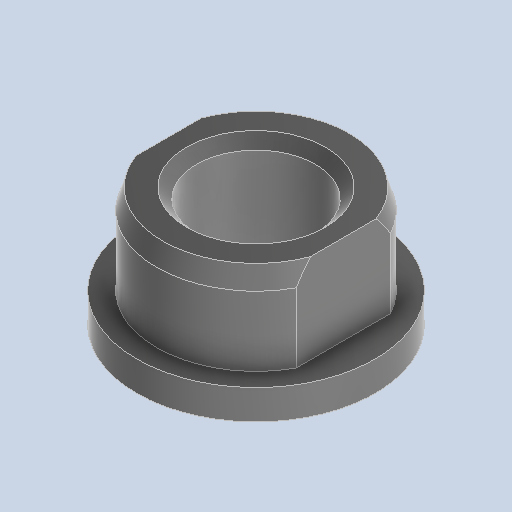
# Autodesk Inventor part: LED-0606
Saved by Autodesk Inventor 2024.2 (Build 282272000, 272)
## iProperties
Created: 2024-01-03
Part Number: LED-0606
Material: Acetal Resin, Black
Document SubType Name: Modeling
Designer: Masato Kubotera
Density: 1.425 g/cm^3
Appearance: Smooth - Black
Catalog Web Link: https://jp.misumi-ec.com/vona2/detail/221000090992/?ProductCode=LED-0606
Vendor: OILES
Mass: 0.469493 g
Surface Area: 4.64015 cm^2
Volume: 0.329469 cm^3
Author: Masato Kubotera
Autodesk Inventor part; units mm, degrees
ref_plane "YZ Plane" through (0, 0, 0) normal (1, 0, 0) x (0, 1, 0)
ref_plane "XZ Plane" through (0, 0, 0) normal (0, 1, 0) x (-1, 0, 0)
ref_plane "XY Plane" through (0, 0, 0) normal (0, 0, 1) x (1, 0, 0)
sketch "Sketch1" plane through (0, 0, 0) normal (0, 1, 0) x (-1, 0, 0)
  line L0 (0, 0) -> (0, 6)
  line L1 (-3, 0) -> (-3, 6)
  line L2 (-3, 6) -> (-5, 6)
  line L3 (-5, 6) -> (-5, 1.5)
  line L4 (-5, 1.5) -> (-6, 1.5)
  line L5 (-6, 1.5) -> (-6, 0)
  line L6 (-6, 0) -> (-3, 0)
  dimension "InsideDiameter" = 6
  dimension "OuterDiameter" = 10
  dimension "FlangeDiameter" = 12
  dimension "FlangeThickness" = 1.5
  dimension "Length" = 6
  constraints: 14 end point, 4 vertical, 3 horizontal, 2 point on line
  measures "InsideDiameter" diameter of L1 L0
  measures "OuterDiameter" diameter of L3 L0
  measures "FlangeDiameter" diameter of L5 L0
  measures "FlangeThickness" distance of L4.end L5.end
  measures "Length" distance of L1.start L1.end
revolve "Revolution1" add sketch "Sketch1" angle 360 about axis through (0, 0, 0) along (0, 0, 1)
chamfer "Chamfer1" distance 0.3 angle 45 1 edges at (-3, 0, 0)
chamfer "Chamfer2" distance 0.5 angle 45 1 edges at (-3, 0, 6)
chamfer "Chamfer3" distance 0.3 distance2 1 1 edges at (-5, 0, 6) measured on face at (4.4516, -0.3989, 6)
sketch "Sketch2" plane through (0, 0, 6) normal (0, 0, 1) x (1, 0, 0)
  circle A0 centre (0, 0) radius 5 projected
  line L0 (-2.3749, -4.4) -> (2.3749, -4.4)
  line L1 (-5, 0) -> (5, 0) construction
  line L2 (-2.3749, 4.4) -> (2.3749, 4.4)
  dimension "Width" = 8.8
  constraints: 6 end point, 6 point on circle, 3 horizontal, 1 midpoint, 1 other
  measures "Width" distance between parallel lines of L2 L0
extrude "Extrusion1" cut sketch "Sketch2" against normal up to surface (4.5 mm away) contours L2 A0 | A0 L0
body "Solid1"
